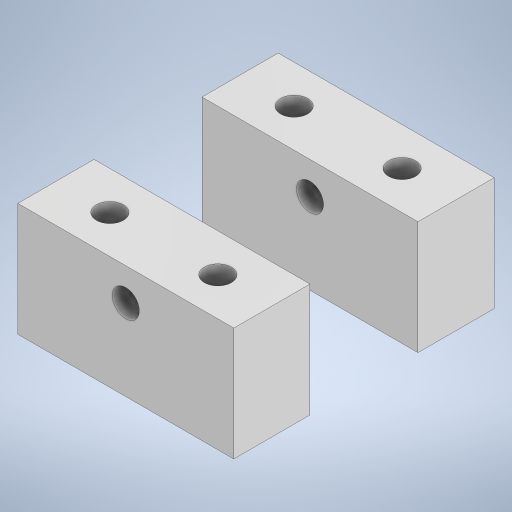
# Autodesk Inventor part: linac_lower_ax_2020_mnt
Saved by Autodesk Inventor 2024 (Build 280153000, 153)
## iProperties
Created: 2025-12-26
Part Number: linac_lower_ax_2020_mnt
Material: PET Plastic
Document SubType Name: Modeling
Designer: schar
Density: 1.541 g/cm^3
Appearance: Polycarbonate - Clear
Author: schar
Autodesk Inventor part; units mm, degrees
ref_plane "Work Plane1" through (-20, 5, 54.056) normal (0, 1, 0) x (1, 0, 0)
sketch "Sketch2" plane through (-20, 5, 54.056) normal (0, 1, 0) x (1, 0, 0)
  point P0 (20, 54.056)
ref_plane "Work Plane2" through (-20, 5, 54.056) normal (0, 1, 0) x (1, 0, 0)
sketch "Sketch3" plane through (-20, 5, 54.056) normal (0, 1, 0) x (1, 0, 0)
  circle A0 centre (10, 71.112) radius 2.5 projected
  circle A1 centre (10, 37) radius 2.5 projected
  line L0 (10, 71.112) -> (10, 64.056)
  line L1 (10, 64.056) -> (0, 64.056)
  line L2 (0, 108.112) -> (0, 0) projected
  line L3 (40, 0) -> (40, 108.112) projected
  line L4 (0, 64.056) -> (40, 64.056)
  line L5 (40, 64.056) -> (40, 78.168)
  line L6 (40, 78.168) -> (0, 78.168)
  line L7 (0, 78.168) -> (0, 64.056)
  line L8 (20, 54.056) -> (40, 54.056)
  line L9 (0, 0) -> (0, 108.112)
  line L10 (40, 108.112) -> (40, 0)
  line L11 (0, 44.056) -> (40, 44.056)
  line L12 (40, 29.944) -> (0, 29.944)
  circle A2 centre (30, 71.112) radius 2.5 projected
  circle A3 centre (30, 71.112) radius 2.5
  circle A4 centre (30, 37) radius 2.5 projected
  circle A5 centre (30, 37) radius 2.5
  dimension "d1" = 7.056
  dimension "d2" = 14.112
  constraints: 22 end point, 8 symmetric about line, 4 point on line, 2 centre point, 2 coincident, 2 horizontal, 2 parallel, 1 midpoint, 1 perpendicular, 1 vertical
  measures "d1" distance of L0.start L0.end
  measures "d2" distance of L5.end L4.end
extrude "Extrusion1" add sketch "Sketch3" along normal blind 25 contours L1 L2 L6 L3 L4 | L11 L3 L12 L2
sketch "Sketch4" plane through (-20, 5, 24.112) normal (0, 0, 1) x (1, 0, 0)
  line L0 (40, 25) -> (0, 25) projected
  line L1 (0, 25) -> (20, 25)
  line L2 (20, 25) -> (20, 15)
  circle A0 centre (20, 15) radius 2.5
  point P0 (20, -5)
  dimension "d5" = 10
  dimension "d6" = 5
  constraints: 4 end point, 1 centre point, 1 coincident, 1 midpoint, 1 perpendicular
  measures "d5" distance of L1.end L2.end
  measures "d6" diameter of A0
extrude "Extrusion2" cut sketch "Sketch4" against normal through all
ref_plane "Work Plane3" through (-20, 30, 54.056) normal (0, 1, 0) x (1, 0, 0)
sketch "Sketch6" plane through (-20, 30, 54.056) normal (0, 1, 0) x (1, 0, 0)
  line L0 (55.7566, 97.8205) -> (-24.6957, 97.8205)
  line L1 (-24.6957, 97.8205) -> (-24.6957, 9.1741)
  line L2 (-24.6957, 9.1741) -> (55.7566, 9.1741)
  line L3 (55.7566, 9.1741) -> (55.7566, 97.8205)
  point P0 (20, 54.056)
  constraints: 8 end point, 2 parallel, 1 horizontal, 1 perpendicular
extrude "Extrusion4" cut sketch "Sketch6" against normal blind 4
body "Solid1"
